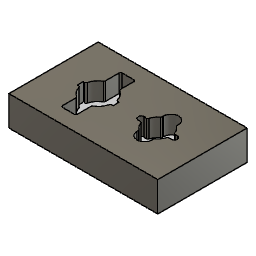
C64 C128 Amiga Mitsumi Fixture v21 (Autodesk Fusion 360 archive; units mm, degrees)
design "C64 C128 Amiga Mitsumi Fixture" references "Mitsumi PCB"
Autodesk Fusion 360 part; units mm, degrees
sketch "Block" plane through (0, 0, 0) normal (0, 1, 0) x (1, 0, 0)
  line L0 (0, 0) -> (50, 0)
  line L1 (50, 0) -> (50, -30)
  line L2 (50, -30) -> (0, -30)
  line L3 (0, -30) -> (0, 0)
  dimension "d1" = 50
  dimension "d2" = 30
  constraint horizontal L0
  constraint vertical L1
  constraint horizontal L2
  constraint vertical L3
  constraint coincident L0.start L3.end
  measures "d1" distance of L0.start L0.end
  measures "d2" distance of L0.start L2.end
extrude "Block (1)" add sketch "Block" along normal blind 10 makes body 1
shell "Hollow Out" thickness 6 removed faces 1 at (16.6667, 0, 10) on bodies 1
sketch "PCB Recess" plane through (0, 0, 0) normal (0, -1, 0) x (1, 0, 0)
  line L0 (6, 6) -> (6, 24)
  line L1 (6, 24) -> (44, 24)
  line L2 (44, 24) -> (44, 6)
  line L3 (44, 6) -> (6, 6)
  line L4 (50, 30) -> (0, 30)
  line L5 (0, 30) -> (0, 0)
  line L6 (0, 0) -> (50, 0)
  line L7 (50, 0) -> (50, 30)
  line L8 (48.5, 1.5) -> (1.5, 1.5)
  line L9 (1.5, 1.5) -> (1.5, 28.5)
  line L10 (1.5, 28.5) -> (48.5, 28.5)
  line L11 (48.5, 28.5) -> (48.5, 1.5)
  dimension "d87" = 27
  dimension "d88" = 47
  dimension "d95" = 1.5
  dimension "d96" = 1.5
  constraint parallel L3 L8
  constraint parallel L0 L9
  constraint parallel L1 L10
  constraint parallel L2 L11
  measures "d87" distance of L8 L10
  measures "d88" distance of L9 L11
  measures "d95" distance of L4 L10
  measures "d96" distance of L5 L9
extrude "PCB Recess (1)" cut sketch "PCB Recess" against normal blind 4 contours L0 L1 L2 L3 | L8 L9 L10 L11 bodies 1
sketch "Key Profiles" plane through (0, 10, 0) normal (0, 1, 0) x (-1, 0, 0)
  line L0 (0, 30) -> (-50, 30)
  line L1 (-50, 30) -> (-50, 0)
  line L2 (-50, 0) -> (0, 0)
  line L3 (0, 0) -> (0, 30)
  line L4 (-15, 0) -> (-15, 30) construction
  line L5 (-35, 0) -> (-35, 30) construction
  arc A0 (-40.625, 16) -> (-40.625, 14) centre (-40.625, 15) ccw
  arc A1 (-29.375, 14) -> (-29.375, 16) centre (-29.375, 15) ccw
  arc A2 (-37.4995, 10.5005) -> (-32.4995, 10.4995) centre (-34.9995, 10.5) ccw
  arc A3 (-32.5001, 19.4994) -> (-37.5001, 19.5006) centre (-35.0001, 19.5) ccw
  line L6 (-12.5, 5) -> (-17.5, 5)
  line L7 (-12.5, 25) -> (-17.4801, 25)
  line L8 (-12.5, 5) -> (-12.5, 25)
  line L9 (-17.4801, 25) -> (-17.5, 5)
  line L10 (-29.375, 14) -> (-40.625, 14)
  line L11 (-29.375, 16) -> (-40.625, 16)
  line L12 (-32.4995, 10.4995) -> (-32.5001, 19.4994)
  line L13 (-37.4995, 10.5005) -> (-37.5001, 19.5006)
  circle A4 centre (-35, 15) radius 4.5
  circle A5 centre (-15, 15) radius 5.25
  line L14 (-9, 14) -> (-21, 14)
  line L15 (-21, 14) -> (-21, 16)
  line L16 (-21, 16) -> (-9, 16)
  line L17 (-9, 16) -> (-9, 14)
  dimension "d9" = 15
  dimension "d10" = 15
  dimension "d16" = 2
  dimension "d17" = 2
  dimension "d120" = 11.25
  dimension "d121" = 15
  dimension "d122" = 15
  dimension "d124" = 2.5
  dimension "d125" = 2.5
  dimension "d126" = 9
  dimension "d127" = 9
  dimension "d128" = 4.5
  dimension "d129" = 10.5
  dimension "d130" = 20
  dimension "d131" = 5
  dimension "d134" = 10
  dimension "d135" = 2.5
  dimension "d146" = 12
  dimension "d147" = 2
  dimension "d148" = 1
  dimension "d149" = 6
  constraint coincident L2 L4.start
  constraint coincident L0 L4.end
  constraint perpendicular L0 L4
  constraint coincident L2 L5.start
  constraint coincident L0 L5.end
  constraint perpendicular L0 L5
  constraint perpendicular L2 L8
  constraint tangent A0 L10
  constraint tangent A0 L11
  constraint midpoint L5 A4.centre
  constraint midpoint L4 A5.centre
  constraint horizontal L14
  constraint vertical L15
  constraint horizontal L16
  constraint vertical L17
  measures "d9" distance of L3 L4
  measures "d10" distance of L1 L5
  measures "d16" diameter of A1
  measures "d17" diameter of A0
  measures "d120" distance of A1.centre A0.centre
  measures "d121" distance of L2 A0.centre
  measures "d122" distance of L2 A1.centre
  measures "d124" radius of A2
  measures "d125" radius of A3
  measures "d126" diameter of A4
  measures "d127" vertical distance of A2.centre A3.centre
  measures "d128" vertical distance of A2.centre A4.centre
  measures "d129" diameter of A5
  measures "d130" distance of L6 L7
  measures "d131" distance of L6.start L6.end
  measures "d134" distance of L6 A5.centre
  measures "d135" distance of L8 A5.centre
  measures "d146" distance of L14.start L14.end
  measures "d147" distance of L14.start L16.end
  measures "d148" distance of A5.centre L14
  measures "d149" distance of A5.centre L17
extrude "Key Profiles (1)" cut sketch "Key Profiles" against normal through all contours A0 L10 L11 A4 | L11 L13 A4 | L10 L11 L13 A4 | L10 L13 A4 | L11 L12 L13 A4 | L10 L11 L12 L13 | A3 L12 L13 A4 | L10 L12 L13 A4 | A2 L12 L13 A4 | L11 L12 A4 | L10 L11 L12 A4 | L10 L12 A4 | A1 L10 L11 A4 | L6 L8 L9 A5 | L8 L9 A5 L14 | L8 A5 L14 | L9 A5 L14 | L8 L9 L14 L16 | L8 A5 L14 L16 | A5 L14 L16 L17 | L9 A5 L14 L16 | A5 L14 L15 L16 | L8 L9 A5 L16 | L8 A5 L16 | L9 A5 L16 | L7 L8 L9 A5 bodies 1
fillet "Fillet3" radius 0.5 8 edges at (37.4996, 7, 11.2581) (39.3875, 7, 14) (32.4996, 7, 11.2586) (30.6125, 7, 14) (30.6125, 7, 16) (32.5001, 7, 18.7417) (39.3875, 7, 16) (37.5001, 7, 18.7416) on bodies 1
fillet "Fillet3" radius 0.5 12 edges at (12.5, 7, 10.3835) (9.8461, 7, 14) (17.4946, 7, 10.3806) (20.1539, 7, 14) (12.5, 7, 5) (17.5, 7, 5) (20.1539, 7, 16) (17.4854, 7, 19.6244) (17.4801, 7, 25) (12.5, 7, 25) (12.5, 7, 19.6165) (9.8461, 7, 16) on bodies 1
sketch "Screw_Holes" plane through (0, 4, 0) normal (0, -1, 0) x (1, 0, 0)
  line L0 (17.5, 10.0946) -> (17.5, 5.25)
  arc A0 (21, 15.75) -> (20.75, 16) centre (20.75, 15.75) ccw
  line L1 (21, 15.75) -> (21, 14.25)
  arc A1 (20.75, 14) -> (21, 14.25) centre (20.75, 14.25) ccw
  line L2 (20.75, 14) -> (20.3561, 14)
  arc A2 (20.3561, 14) -> (20.1126, 13.8068) centre (20.3561, 13.75) ccw
  arc A3 (17.7391, 10.5212) -> (20.1126, 13.8068) centre (15, 15) ccw
  arc A4 (17.7391, 10.5212) -> (17.5, 10.0946) centre (18, 10.0946) ccw
  arc A5 (17.5, 19.9054) -> (17.7391, 19.4788) centre (18, 19.9054) ccw
  arc A6 (20.1126, 16.1932) -> (17.7391, 19.4788) centre (15, 15) ccw
  arc A7 (20.1126, 16.1932) -> (20.3561, 16) centre (20.3561, 16.25) ccw
  arc A8 (17.25, 5) -> (17.5, 5.25) centre (17.25, 5.25) ccw
  line L3 (17.25, 5) -> (12.75, 5)
  arc A9 (12.5, 5.25) -> (12.75, 5) centre (12.75, 5.25) ccw
  line L4 (12.5, 5.25) -> (12.5, 10.0946)
  arc A10 (12.5, 10.0946) -> (12.2609, 10.5212) centre (12, 10.0946) ccw
  arc A11 (9.8874, 13.8068) -> (12.2609, 10.5212) centre (15, 15) ccw
  arc A12 (9.8874, 13.8068) -> (9.6439, 14) centre (9.6439, 13.75) ccw
  arc A13 (9, 14.25) -> (9.25, 14) centre (9.25, 14.25) ccw
  line L5 (9, 14.25) -> (9, 15.75)
  arc A14 (9.25, 16) -> (9, 15.75) centre (9.25, 15.75) ccw
  line L6 (9.25, 16) -> (9.6439, 16)
  arc A15 (9.6439, 16) -> (9.8874, 16.1932) centre (9.6439, 16.25) ccw
  arc A16 (12.2609, 19.4788) -> (9.8874, 16.1932) centre (15, 15) ccw
  arc A17 (12.2609, 19.4788) -> (12.5, 19.9054) centre (12, 19.9054) ccw
  arc A18 (12.75, 25) -> (12.5, 24.75) centre (12.75, 24.75) ccw
  line L7 (12.75, 25) -> (17.25, 25)
  arc A19 (17.5, 24.75) -> (17.25, 25) centre (17.25, 24.75) ccw
  line L8 (48.5, 28.5) -> (1.5, 28.5)
  line L9 (1.5, 28.5) -> (1.5, 1.5)
  line L10 (1.5, 1.5) -> (48.5, 1.5)
  line L11 (48.5, 1.5) -> (48.5, 28.5)
  line L12 (9.6439, 14) -> (9.25, 14)
  line L13 (12.5, 19.9054) -> (12.5, 24.75)
  line L14 (17.5, 24.75) -> (17.5, 19.9054)
  line L15 (20.3561, 16) -> (20.75, 16)
  line L16 (37.5, 11.2583) -> (37.5, 10.5)
  arc A20 (32.5, 10.5) -> (37.5, 10.5) centre (35, 10.5) ccw
  line L17 (32.5, 10.5) -> (32.5, 11.2583)
  arc A21 (30.6125, 14) -> (32.5, 11.2583) centre (35, 15) ccw
  line L18 (30.6125, 14) -> (29.375, 14)
  arc A22 (29.375, 16) -> (29.375, 14) centre (29.375, 15) ccw
  line L19 (29.375, 16) -> (30.6125, 16)
  arc A23 (32.5, 18.7417) -> (30.6125, 16) centre (35, 15) ccw
  line L20 (32.5, 18.7417) -> (32.5, 19.5)
  arc A24 (37.5, 19.5) -> (32.5, 19.5) centre (35, 19.5) ccw
  line L21 (37.5, 19.5) -> (37.5, 18.7417)
  arc A25 (39.3875, 16) -> (37.5, 18.7417) centre (35, 15) ccw
  line L22 (39.3875, 16) -> (40.625, 16)
  arc A26 (40.625, 14) -> (40.625, 16) centre (40.625, 15) ccw
  line L23 (40.625, 14) -> (39.3875, 14)
  arc A27 (37.5, 11.2583) -> (39.3875, 14) centre (35, 15) ccw
  point P0 (6, 24)
  point P1 (44, 23.75)
  point P2 (44, 5.75)
  point P3 (6, 6)
  dimension "d45" = 38
  dimension "d46" = 38
  dimension "d47" = 18
  dimension "d48" = 18
  measures "d45" horizontal distance of P0 P1
  measures "d46" horizontal distance of P2 P3
  measures "d47" distance of P0 P3
  measures "d48" distance of P1 P2
hole "PCB Mounting Holes" [rolled back] hole depth 4 hole diameter 2 tip angle 118
sketch "Lead Exit" plane through (50, 0, 0) normal (1, 0, 0) x (0, 0, -1)
  line L0 (-30, 0) -> (0, 0)
  line L1 (0, 0) -> (0, 10)
  line L2 (0, 10) -> (-30, 10)
  line L3 (-30, 10) -> (-30, 0)
  line L4 (-17, 0) -> (-13, 0)
  line L5 (-13, 0) -> (-13, 1.5)
  line L6 (-13.5, 2) -> (-16.5, 2)
  line L7 (-17, 1.5) -> (-17, 0)
  arc A0 (-16.5, 2) -> (-17, 1.5) centre (-16.5, 1.5) ccw
  arc A1 (-13, 1.5) -> (-13.5, 2) centre (-13.5, 1.5) ccw
  dimension "d56" = 4
  dimension "d57" = 30
  dimension "d58" = 13
  dimension "d59" = 0.5
  constraint horizontal L4
  constraint vertical L5
  constraint horizontal L6
  constraint vertical L7
  constraint coincident L0 L4.start
  constraint tangent L6 A0
  constraint tangent L7 A0
  constraint tangent L6 A1
  constraint tangent L5 A1
  constraint equal A0 A1
  measures "d56" distance of L4.start L4.end
  measures "d57" distance of L1.end L2.end
  measures "d58" distance of L3 L7
  measures "d59" radius of A0
extrude "Lead Exit (1)" [rolled back] along distance -4 taper angle 0
sketch "Lead clearance" plane through (0, 4, 0) normal (0, -1, 0) x (1, 0, 0)
  line L0 (17.5, 10.0946) -> (17.5, 5.25)
  arc A0 (21, 15.75) -> (20.75, 16) centre (20.75, 15.75) ccw
  line L1 (21, 15.75) -> (21, 14.25)
  arc A1 (20.75, 14) -> (21, 14.25) centre (20.75, 14.25) ccw
  line L2 (20.75, 14) -> (20.3561, 14)
  line L3 (48.5, 18) -> (44.5, 18)
  line L4 (44, 17.5) -> (44, 12.5)
  line L5 (44.5, 12) -> (48.5, 12)
  line L6 (48.5, 12) -> (48.5, 18)
  arc A2 (44.5, 18) -> (44, 17.5) centre (44.5, 17.5) ccw
  arc A3 (44, 12.5) -> (44.5, 12) centre (44.5, 12.5) ccw
  arc A4 (20.3561, 14) -> (20.1126, 13.8068) centre (20.3561, 13.75) ccw
  arc A5 (17.7391, 10.5212) -> (20.1126, 13.8068) centre (15, 15) ccw
  arc A6 (17.7391, 10.5212) -> (17.5, 10.0946) centre (18, 10.0946) ccw
  arc A7 (17.5, 19.9054) -> (17.7391, 19.4788) centre (18, 19.9054) ccw
  arc A8 (20.1126, 16.1932) -> (17.7391, 19.4788) centre (15, 15) ccw
  arc A9 (20.1126, 16.1932) -> (20.3561, 16) centre (20.3561, 16.25) ccw
  circle A10 centre (44, 23.75) radius 1
  circle A11 centre (6, 6) radius 1
  circle A12 centre (6, 24) radius 1
  circle A13 centre (44, 5.75) radius 1
  arc A14 (17.25, 5) -> (17.5, 5.25) centre (17.25, 5.25) ccw
  line L7 (17.25, 5) -> (12.75, 5)
  arc A15 (12.5, 5.25) -> (12.75, 5) centre (12.75, 5.25) ccw
  line L8 (12.5, 5.25) -> (12.5, 10.0946)
  arc A16 (12.5, 10.0946) -> (12.2609, 10.5212) centre (12, 10.0946) ccw
  arc A17 (9.8874, 13.8068) -> (12.2609, 10.5212) centre (15, 15) ccw
  arc A18 (9.8874, 13.8068) -> (9.6439, 14) centre (9.6439, 13.75) ccw
  arc A19 (9, 14.25) -> (9.25, 14) centre (9.25, 14.25) ccw
  line L9 (9, 14.25) -> (9, 15.75)
  arc A20 (9.25, 16) -> (9, 15.75) centre (9.25, 15.75) ccw
  line L10 (9.25, 16) -> (9.6439, 16)
  arc A21 (9.6439, 16) -> (9.8874, 16.1932) centre (9.6439, 16.25) ccw
  arc A22 (12.2609, 19.4788) -> (9.8874, 16.1932) centre (15, 15) ccw
  arc A23 (12.2609, 19.4788) -> (12.5, 19.9054) centre (12, 19.9054) ccw
  arc A24 (12.75, 25) -> (12.5, 24.75) centre (12.75, 24.75) ccw
  line L11 (12.75, 25) -> (17.25, 25)
  arc A25 (17.5, 24.75) -> (17.25, 25) centre (17.25, 24.75) ccw
  line L12 (48.5, 28.5) -> (1.5, 28.5)
  line L13 (1.5, 28.5) -> (1.5, 1.5)
  line L14 (1.5, 1.5) -> (48.5, 1.5)
  line L15 (48.5, 1.5) -> (48.5, 28.5)
  line L16 (9.6439, 14) -> (9.25, 14)
  line L17 (12.5, 19.9054) -> (12.5, 24.75)
  line L18 (17.5, 24.75) -> (17.5, 19.9054)
  line L19 (20.3561, 16) -> (20.75, 16)
  line L20 (37.5, 11.2583) -> (37.5, 10.5)
  arc A26 (32.5, 10.5) -> (37.5, 10.5) centre (35, 10.5) ccw
  line L21 (32.5, 10.5) -> (32.5, 11.2583)
  arc A27 (30.6125, 14) -> (32.5, 11.2583) centre (35, 15) ccw
  line L22 (30.6125, 14) -> (29.375, 14)
  arc A28 (29.375, 16) -> (29.375, 14) centre (29.375, 15) ccw
  line L23 (29.375, 16) -> (30.6125, 16)
  arc A29 (32.5, 18.7417) -> (30.6125, 16) centre (35, 15) ccw
  line L24 (32.5, 18.7417) -> (32.5, 19.5)
  arc A30 (37.5, 19.5) -> (32.5, 19.5) centre (35, 19.5) ccw
  line L25 (37.5, 19.5) -> (37.5, 18.7417)
  arc A31 (39.3875, 16) -> (37.5, 18.7417) centre (35, 15) ccw
  line L26 (39.3875, 16) -> (40.625, 16)
  arc A32 (40.625, 14) -> (40.625, 16) centre (40.625, 15) ccw
  line L27 (40.625, 14) -> (39.3875, 14)
  arc A33 (37.5, 11.2583) -> (39.3875, 14) centre (35, 15) ccw
  point P0 (44, 18)
  point P1 (50, 0)
  point P2 (50, 30)
  dimension "d62" = 4.5
  dimension "d63" = 6
  dimension "d64" = 30
  dimension "d65" = 12
  dimension "d66" = 0.5
  dimension "d73" = 1.5
  dimension "d74" = 2
  constraint horizontal L3
  constraint vertical L4
  constraint horizontal L5
  constraint vertical L6
  constraint coincident P0 L3
  constraint coincident P0 L4
  constraint tangent L3 A2
  constraint tangent L4 A2
  constraint tangent L4 A3
  constraint tangent L5 A3
  constraint equal A2 A3
  measures "d62" distance of L3.start P0
  measures "d63" distance of L3.start L5.end
  measures "d64" distance of P1 P2
  measures "d65" distance of L3 P2
  measures "d66" radius of A2
  measures "d73" distance of L6 P2
extrude "Lead clearance (1)" [rolled back] along distance -2 taper angle 0
copy_body "Body->Comp1" bodies 1 removing the originals makes body 2 in component "Component"
equation "d1 = Block_Width"
equation "d2 = Block_Height"
equation "d10 = d9"
equation "d16 = Amiga_Stem_H_Height"
equation "d17 = Amiga_Stem_H_Height"
equation "d46 = d45"
equation "d48 = d47"
equation "d58 = ( 30.00 mm - d56 ) / 2"
equation "d65 = ( 30.00 mm - d63 ) / 2"
equation "d73 = Wall"
equation "d87 = PCB_Height"
equation "d88 = PCB_Width"
equation "PCB_Height = 27 mm"
equation "PCB_Width = 47 mm"
equation "Block_Width = 50 mm"
equation "Block_Height = 30 mm"
equation "Wall = ( Block_Width - PCB_Width ) / 2"
equation "d95 = Wall"
equation "d96 = Wall"
equation "Amiga_Stem_V_Width = 5 mm"
equation "Amiga_Stem_V_Height = 9 mm"
equation "Amiga_Stem_H_Width = 11.25 mm"
equation "Amiga_Stem_H_Height = 2 mm"
equation "Amiga_Stem_Hole_Dia = 9 mm"
equation "d120 = Amiga_Stem_H_Width"
equation "d122 = d121"
equation "d124 = Amiga_Stem_V_Width / 2"
equation "d125 = Amiga_Stem_V_Width / 2"
equation "d126 = Amiga_Stem_Hole_Dia"
equation "d127 = Amiga_Stem_V_Height"
equation "d128 = Amiga_Stem_V_Height / 2"
equation "d129 = C64_Stem_Hole_Dia"
equation "d130 = C64_Stem_V_Height"
equation "d131 = C64_Stem_V_Width"
equation "d134 = C64_Stem_V_Height / 2"
equation "d135 = C64_Stem_V_Width / 2"
equation "C64_Stem_V_Width = 5 mm"
equation "C64_Stem_V_Height = 20 mm"
equation "C64_Stem_H_Width = 12 mm"
equation "C64_Stem_H_Height = 2 mm"
equation "C64_Stem_Hole_Dia = 10.5 mm"
equation "d146 = C64_Stem_H_Width"
equation "d147 = C64_Stem_H_Height"
equation "d148 = C64_Stem_H_Height / 2"
equation "d149 = C64_Stem_H_Width / 2"
